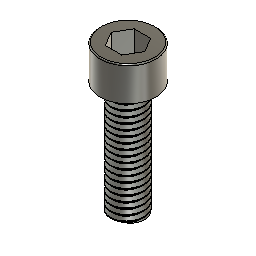
Touchprobe (Autodesk Fusion 360 archive; units mm, degrees)
design "M6x20"
Autodesk Fusion 360 part; units mm, degrees
sketch "Skizze1" plane through (0, 0, 0) normal (0, 1, 0) x (1, 0, 0)
  line L0 (0, -88.5326) -> (0, 41.4674) construction
  line L1 (0, 27) -> (-3, 27)
  line L2 (-3, 27) -> (-3, 7)
  line L3 (-3, 7) -> (-4.9, 7)
  line L4 (-4.9, 7) -> (-4.9, 1)
  line L5 (-4.9, 1) -> (0, 1)
  line L6 (0, 27) -> (0, 1)
  dimension "d1" = 3
  dimension "d2" = 20
  dimension "d4" = 6
  dimension "d5" = 1
  dimension "d7" = 4.9
  constraint vertical L0
  constraint coincident L0 L1.start
  constraint perpendicular L0 L1
  constraint perpendicular L1 L2
  constraint perpendicular L2 L3
  constraint perpendicular L3 L4
  constraint perpendicular L0 L5
  constraint coincident L0 L5.end
  constraint coincident origin L0
  measures "d1" distance of L1.start L1.end
  measures "d2" distance of L1.end L2.end
  measures "d4" distance of L3.end L4.end
  measures "d5" distance of origin L5
  measures "d7" distance of L4 L6
revolve "Drehen1" add sketch "Skizze1" angle 360 about axis through (0, 0, 88.5326) along (0, 0, -1)
sketch "Skizze2" plane through (0, 0, -1) normal (0, 0, 1) x (-1, 0, 0)
  circle A0 centre (0, 0) radius 4.9
  line L0 (1.4722, -2.55) -> (2.9445, 0)
  line L1 (2.9445, 0) -> (1.4722, 2.55)
  line L2 (1.4722, 2.55) -> (-1.4722, 2.55)
  line L3 (-1.4722, 2.55) -> (-2.9445, 0)
  line L4 (-2.9445, 0) -> (-1.4722, -2.55)
  line L5 (-1.4722, -2.55) -> (1.4722, -2.55)
  dimension "d8" = 2.55
  constraint coincident A0.centre origin
  measures "d8" distance of A0.centre L5
extrude "Extrusion1" cut sketch "Skizze2" against normal blind 4.2 contours L0 L1 L2 L3 L4 L5
fillet "Abrundung1" radius 0.2 1 edges at (-4.5684, 1.7719, -1)
thread "Gewinde1" "ISO Metric profile 6.0 M6x1 6g" major diameter 5.884 minor diameter 4.7435 pitch 1 angle 60 modelled right hand crest width 0.1444 on face at (-2.9851, -0.2987, -13.6667) crest through (-2.942, 0, -6.75)
equation "d7 = ( 9.8 / 2 ) * 1 mm"
equation "d8 = ( 5.1 / 2 ) * 1 mm"

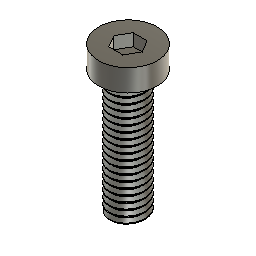
design "m3_x20_schraube"
Autodesk Fusion 360 part; units mm, degrees
sketch "Skizze1" plane through (0, 0, 0) normal (0, 1, 0) x (1, 0, 0)
  line L0 (0, -45) -> (0, 55) construction
  line L1 (0, 15.8) -> (0, 14)
  line L2 (-2.4, 14) -> (0, 14)
  line L3 (-1.519, 15.8) -> (-2.4, 15.8)
  line L4 (-2.4, 15.8) -> (-2.4, 14)
  line L5 (-1.519, 15.8) -> (0, 15.8)
  dimension "d2" = 1.8
  dimension "d3" = 2.4
  constraint vertical L0
  constraint coincident L0 L1.end
  constraint perpendicular L1 L2
  constraint parallel L2 L3
  constraint perpendicular L2 L4
  constraint coincident L0 L1.start
  constraint perpendicular L1 L5
  measures "d2" distance of L2.start L3.end
  measures "d3" distance of L1.end L2.start
revolve "Drehen1" add sketch "Skizze1" angle 360 about axis through (0, 0, 45) along (0, 0, -1) makes body 1
sketch "Skizze2" plane through (0, 0, -14) normal (0, 0, 1) x (-1, 0, 0)
  circle A0 centre (0, 0) radius 2.4
  line L0 (0, -1.7113, -0.988) -> (0, 0, -1.9761)
  line L1 (0, 0, -1.9761) -> (0, 1.7113, -0.988)
  line L2 (0, 1.7113, -0.988) -> (0, 1.7113, 0.988)
  line L3 (0, 1.7113, 0.988) -> (0, 0, 1.9761)
  line L4 (0, 0, 1.9761) -> (0, -1.7113, 0.988)
  line L5 (0, -1.7113, 0.988) -> (0, -1.7113, -0.988)
  line L6 (0.5774, -1) -> (1.1547, 0)
  line L7 (1.1547, 0) -> (0.5774, 1)
  line L8 (0.5774, 1) -> (-0.5774, 1)
  line L9 (-0.5774, 1) -> (-1.1547, 0)
  line L10 (-1.1547, 0) -> (-0.5774, -1)
  line L11 (-0.5774, -1) -> (0.5774, -1)
  dimension "d5" = 2
  constraint coincident A0.centre origin
  measures "d5" distance of L8 L11
extrude "Extrusion1" cut sketch "Skizze2" against normal blind 1 contours L6 L7 L8 L9 L10 L11 bodies 1
copy_body "Körper->Berechn1" bodies 1 removing the originals makes body 2 in component "Component"
sketch "Skizze3" plane through (0, 0, -15.8) normal (0, 0, -1) x (1, 0, 0)
  circle A0 centre (0, 0) radius 2.4
  circle A1 centre (0, 0) radius 1.5
  dimension "d8" = 3
  constraint coincident A0.centre A1.centre
  measures "d8" diameter of A1
extrude "Extrusion1'" add sketch "Skizze3" along normal blind 10 contours A1 bodies 2 in component "Component"
thread "Gewinde1" "ISO Metric profile 3.0 M3x0.5 6g" major diameter 2.927 minor diameter 2.3555 pitch 0.5 angle 60 modelled right hand crest width 0.0713 on face at (1.4981, 0.0748, -22.4667) crest through (1.4635, 0, -15.675) on bodies 2 in component "Component"
component "Component" placed x (1, 0, 0) y (0, 1, 0) z (0, 0, 1) at (0, 0, 0)
